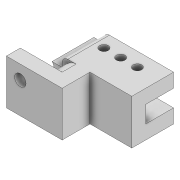
# Autodesk Inventor part: Bending_hinge_p2
Saved by Autodesk Inventor 2022 (Build 260153000, 153)
## iProperties
Created: 2022-07-29
Part Number: Bending_hinge_p2
Material: Generic
Document SubType Name: Modeling
Designer: dell
Density: 1 g/cm^3
Appearance: Default
Author: dell
Autodesk Inventor part; units mm, degrees
ref_plane "XZ Plane" through (0, 0, 0) normal (0, 1, 0) x (-1, 0, 0)
ref_plane "XY Plane" through (0, 0, 0) normal (0, 0, 1) x (1, 0, 0)
sketch "Sketch2" plane through (0, 0, 0) normal (0, 1, 0) x (-1, 0, 0)
  line L0 (0, 0) -> (30, 0)
  line L1 (30, 0) -> (30, -10)
  line L2 (30, -10) -> (0, -10)
  line L3 (0, -10) -> (0, 0)
  circle A0 centre (10, -5) radius 1.55
  dimension "d0" = 3.1
  dimension "d1" = 10
  dimension "d2" = 5
  dimension "d3" = 30
  dimension "d4" = 10
  constraints: 8 end point, 2 parallel, 1 centre point, 1 horizontal, 1 perpendicular
  measures "d0" diameter of A0
  measures "d1" distance from line of L3 A0.centre
  measures "d2" distance from line of L0 A0.centre
  measures "d3" distance between parallel lines of L3 L1
  measures "d4" distance between parallel lines of L0 L2
extrude "Extrusion1" add sketch "Sketch2" along normal blind 5 contours L0 L1 L2 L3 | A0
extrude "Extrusion2" cut sketch "Sketch2" along normal blind 10 contours A0
pattern_linear "Rectangular Pattern1" count 3 spacing 6 along (-1, 0, 0) of "Extrusion2"
pattern_linear "Rectangular Pattern2" count 2 spacing 11.1 along (0, -1, 0) of "Extrusion1", "Extrusion2", "Rectangular Pattern1"
sketch "Sketch3" plane through (-30, 0, 0) normal (0, 0, 1) x (1, 0, 0)
  line L0 (0, 0) -> (0, 5) projected
  line L1 (0, 5) -> (30, 5) projected
  line L2 (30, 5) -> (30, 0) projected
  line L3 (30, 0) -> (0, 0) projected
  line L4 (0, -11.1) -> (0, -6.1) projected
  line L5 (0, -6.1) -> (30, -6.1) projected
  line L6 (30, -6.1) -> (30, -11.1) projected
  line L7 (30, -11.1) -> (0, -11.1) projected
  line L8 (0, 5) -> (30, 5) projected
  line L9 (0, 5) -> (30, 5)
  line L10 (30, 5) -> (30, -11.1)
  line L11 (30, -11.1) -> (0, -11.1)
  line L12 (0, -11.1) -> (0, 5)
  circle A0 centre (30, 0) radius 2.05
  line L13 (30, 5) -> (0, 5) projected
  line L14 (25, 5) -> (35, 5)
  line L15 (35, 5) -> (35, -11.1)
  line L16 (35, -11.1) -> (25, -11.1)
  line L17 (25, -11.1) -> (25, 5)
  line L18 (0, -11.1) -> (30, -11.1) projected
  line L19 (15.55, -11.1) -> (12.45, -11.1) projected
  line L20 (25, 5) -> (20, 5)
  line L21 (20, 5) -> (20, -11.1)
  line L22 (20, -11.1) -> (25, -11.1)
  line L23 (25, -11.1) -> (25, 5)
  line L24 (20, 5) -> (15, 5)
  line L25 (15, 5) -> (15, -11.1)
  line L26 (15, -11.1) -> (20, -11.1)
  line L27 (20, -11.1) -> (20, 5)
  dimension "d36" = 4.1
  dimension "d37" = 5
  dimension "d38" = 5
  dimension "d39" = 5
  dimension "d40" = 5
  constraints: 32 end point, 8 parallel, 4 horizontal, 4 perpendicular, 3 point on line, 1 centre point, 1 coincident, 1 collinear
  measures "d36" diameter of A0
  measures "d37" distance from line of L2.end L17
  measures "d38" distance from line of L15 L2.end
  measures "d39" distance between parallel lines of L23 L21
  measures "d40" distance between parallel lines of L21 L25
extrude "Extrusion3" add sketch "Sketch3" along normal blind 5 contours L0 L1 L25 L3 | L3 L25 L5 L12 | L25 L1 L21 L3 | L3 L21 L5 L25 | L5 L25 L7 L4 | L21 L1 L17 L3 | L3 L17 L5 L21 | L5 L21 L7 L25 | L17 L1 L2 A0 L3 | L3 A0 L10 L5 L17 | L5 L17 L7 L21 | A0 L2 L3 | L3 L10 A0 | L5 L6 L7 L17
extrude "Extrusion4" cut sketch "Sketch3" along normal mid plane 100 contours A0 L2 L3 | L3 L10 A0 | L2 A0 L10
extrude "Extrusion5" add sketch "Sketch3" along normal blind 10 contours L25 L1 L21 L3 | L3 L21 L5 L25 | L21 L1 L17 L3 | L3 L17 L5 L21 | L5 L21 L7 L25 | L5 L17 L7 L21
sketch "Sketch5" plane through (-30, 0, 10) normal (0, 0, 1) x (1, 0, 0)
  line L0 (25, 5) -> (25, -11.1) projected
  line L1 (25, -11.1) -> (15, -11.1) projected
  line L2 (15, -11.1) -> (15, 5) projected
  line L3 (15, 5) -> (25, 5) projected
  line L4 (25, 5) -> (35, 5)
  line L5 (35, 5) -> (35, -11.1)
  line L6 (35, -11.1) -> (25, -11.1)
  line L7 (25, -11.1) -> (25, 5)
  arc A0 (30, 2.05) -> (30, -2.05) centre (30, 0) ccw projected
  arc A1 (27.95, 0) -> (30, -2.05) centre (30, 0) ccw projected
  arc A2 (30, 2.05) -> (27.95, 0) centre (30, 0) ccw projected
  circle A3 centre (30, 0) radius 2.05
  point P0 (30, -2.05)
  point P1 (30, 2.05)
  dimension "d41" = 5
  constraints: 8 end point, 2 parallel, 1 centre point, 1 coincident, 1 concentric, 1 horizontal, 1 perpendicular
  measures "d41" distance from line of point (30, 0) L5
extrude "Extrusion8" add sketch "Sketch5" along normal blind 5
ref_plane "Work Plane2" through (20, 0, 0) normal (1, 0, 0) x (0, 1, 0)
mirror "Mirror2" about plane through (20, 0, 0) normal (1, 0, 0) remove original yes
sketch "Sketch6" plane through (40, 5, 5) normal (0, 0, 1) x (1, 0, 0)
  line L0 (5, 0) -> (5, -16.1) projected
  line L1 (0, 0) -> (5, 0) projected
  line L2 (0, -2.95) -> (0, 0) projected
  arc A0 (0, -7.05) -> (0, -2.95) centre (0, -5) ccw projected
  line L3 (0, -16.1) -> (0, -7.05) projected
  line L4 (5, -16.1) -> (0, -16.1) projected
  line L5 (0, -3.5) -> (5, -3.5)
  line L6 (5, 0) -> (5, -16.1) projected
  point P0 (-40, -5)
  point P1 (1.3973, -3.5)
  dimension "d47" = 3.5
  constraints: 2 end point, 1 perpendicular, 1 point on line
  measures "d47" distance between parallel lines of L1 L5
extrude "Extrusion9" cut sketch "Sketch6" against normal blind 100 contours L0 L5 A0 L2 L1
sketch "Sketch7" plane through (45, -11.1, 10) normal (-1, 0, 0) x (0, 0, 1)
  line L0 (-5, 12.6) -> (-5, 0) projected
  line L1 (-5, 0) -> (0, 0) projected
  line L2 (0, 0) -> (0, 16.1) projected
  line L3 (-20, 16.1) -> (0, 16.1) projected
  line L4 (-20, 12.6) -> (-20, 16.1) projected
  line L5 (-5, 12.6) -> (-20, 12.6) projected
  line L6 (-5, 16.1) -> (-5, 0) projected
  line L7 (-5, 12.6) -> (-5, 16.1)
  point P0 (-10, 11.1)
  constraints: 2 end point, 1 vertical
extrude "Extrusion10" cut sketch "Sketch7" against normal blind 1 contours L6 L3 L2 L1 L0
fillet "Fillet1" radius 4 1 edges at (46, 5, 7.5)
fillet "Fillet2" radius 2 1 edges at (45, 5, -2.5)
body "Solid1"
